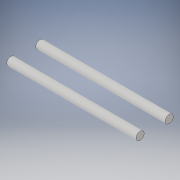
# Autodesk Inventor part: Mounting Rods
Saved by Autodesk Inventor 2019 (Build 230136000, 136)
## iProperties
Created: 2019-10-21
Part Number: Mounting Rods
Material: Generic
Document SubType Name: Modeling
Designer: 19879326
Density: 1 g/cm^3
Appearance: Default
Author: 19879326
Autodesk Inventor part; units mm, degrees
ref_plane "YZ Plane" through (0, 0, 0) normal (1, 0, 0) x (0, 1, 0)
ref_plane "XZ Plane" through (0, 0, 0) normal (0, 1, 0) x (-1, 0, 0)
ref_plane "XY Plane" through (0, 0, 0) normal (0, 0, 1) x (1, 0, 0)
sketch "Sketch1" plane through (0, 0, 0) normal (1, 0, 0) x (0, 1, 0)
  circle A0 centre (0, 45) radius 12.5
  circle A1 centre (0, -45) radius 12.5
  point P0 (0, 0)
  dimension "d0" = 25
  dimension "d1" = 45
  dimension "d2" = 90
  constraints: 2 centre point, 2 vertical alignment, 1 equal radius
  measures "d0" diameter of A0
  measures "d1" distance of point (0, 0) A0.centre
  measures "d2" distance of A1.centre A0.centre
extrude "Extrusion1" add sketch "Sketch1" along normal blind 400
body "Solid1"
